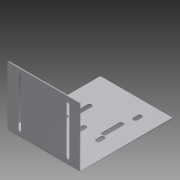
# Autodesk Inventor part: subframe
Saved by Autodesk Inventor 2014 SP2 (Build 180246200, 246)
## iProperties
Created: 2016-05-19
Part Number: subframe
Material: Aluminum 6061
Document SubType Name: Sheet Metal
Designer: cruiser
Density: 2.71 g/cm^3
Sheet Metal Rule: Default_mm
Appearance: Aluminum - Flat
Flat Pattern Width: 13.862 cm
Flat Pattern Length: 6.6 cm
Flat Pattern Area: 91.4895 cm^2
Sheet Metal Width: 138.620 mm
Sheet Metal Length: 66.000 mm
Sheet Metal Area: 9148.948 mm^2
Author: cruiser
Autodesk Inventor part; units mm, degrees
ref_plane "YZ Plane" through (0, 0, 0) normal (1, 0, 0) x (0, 1, 0)
ref_plane "XZ Plane" through (0, 0, 0) normal (0, 1, 0) x (-1, 0, 0)
ref_plane "XY Plane" through (0, 0, 0) normal (0, 0, 1) x (1, 0, 0)
sketch "Sketch1" plane through (0, 0, 0) normal (0, 1, 0) x (-1, 0, 0)
  line L0 (33, -27.5) -> (-33, -27.5)
  line L1 (-33, -27.5) -> (-33, 27.5)
  line L2 (-33, 27.5) -> (33, 27.5)
  line L3 (33, 27.5) -> (33, -27.5)
  line L4 (33, -27.5) -> (-33, 27.5) construction
  line L5 (-33, -27.5) -> (33, 27.5) construction
  point P0 (0, 0)
  dimension "d0" = 66
  dimension "d1" = 55
  measures "d0" distance of L1.end L2.end
  measures "d1" distance of L0.end L1.end
extrude "Plate1" add sketch "Sketch1" along normal blind 0.7937
sketch "Sketch3" plane through (0, 0.7937, 0) normal (0, 1, 0) x (1, 0, 0)
  line L0 (0, 0) -> (-33, 0)
  line L1 (-33, 0) -> (-33, 27.5)
  line L2 (-33, 27.5) -> (0, 27.5)
  line L3 (0, 27.5) -> (0, 0)
  circle A0 centre (-22, 16) radius 1.5
  circle A1 centre (-22, -16) radius 1.5
  circle A2 centre (22, 16) radius 1.5
  circle A3 centre (22, -16) radius 1.5
  line L4 (-22, 11) -> (-22, 21) construction
  line L5 (-20.5, 11) -> (-20.5, 21)
  line L6 (-23.5, 21) -> (-23.5, 11)
  arc A4 (-23.5, 11) -> (-20.5, 11) centre (-22, 11) ccw
  arc A5 (-20.5, 21) -> (-23.5, 21) centre (-22, 21) ccw
  line L7 (20.5, 11) -> (20.5, 21)
  line L8 (23.5, 21) -> (23.5, 11)
  arc A6 (20.5, 11) -> (23.5, 11) centre (22, 11) ccw
  arc A7 (23.5, 21) -> (20.5, 21) centre (22, 21) ccw
  line L9 (-20.5, -11) -> (-20.5, -21)
  line L10 (-23.5, -21) -> (-23.5, -11)
  arc A8 (-20.5, -11) -> (-23.5, -11) centre (-22, -11) ccw
  arc A9 (-23.5, -21) -> (-20.5, -21) centre (-22, -21) ccw
  arc A10 (20.5, -21) -> (23.5, -21) centre (22, -21) ccw
  line L11 (23.5, -21) -> (23.5, -11)
  line L12 (20.5, -11) -> (20.5, -21)
  arc A11 (23.5, -11) -> (20.5, -11) centre (22, -11) ccw
  line L13 (-23.5, 16) -> (-20.5, 16)
  line L14 (-20.5, 16) -> (-20.5, -16)
  line L15 (-20.5, -16) -> (-23.5, -16)
  line L16 (-23.5, -16) -> (-23.5, 16)
  line L17 (20.5, -16) -> (23.5, -16)
  line L18 (23.5, -16) -> (23.5, 16)
  line L19 (23.5, 16) -> (20.5, 16)
  line L20 (20.5, 16) -> (20.5, -16)
  dimension "d22" = 3
  dimension "d23" = 32
  dimension "d24" = 22
  dimension "d48" = 5
  dimension "d49" = 3
  constraints: 44 end point, 21 symmetric about line, 16 point on circle, 11 centre point, 8 parallel, 5 midpoint, 4 tangent, 3 horizontal, 3 perpendicular, 1 horizontal alignment, 11 other
  measures "d22" diameter of A0
  measures "d23" diameter of A0.centre L0
  measures "d24" distance from line of L3 A0.centre
  measures "d48" distance of A0.centre L4.end
  measures "d49" diameter of A5
extrude "Cut1" cut sketch "Sketch3" against normal blind 0.7937 contours L14 A8 L16 L0 | L0 L16 A4 L14 | A4 L6 A0 L5 | L9 A1 L10 A8 | L13 A0 | A0 L6 A5 L5 | A0 L13 | L15 A1 | L9 A9 L10 A1 | A1 L15 | L19 A2 | L8 A6 L7 A2 | A2 L7 A7 L8 | A2 L19 | L18 A11 L20 A6 | L11 A3 L12 A11 | L17 A3 | L11 A10 L12 A3 | A3 L17
sketch "Sketch2" plane through (-33, 0, -26.7063) normal (0, 0, -1) x (-1, 0, 0)
  line L0 (-66, 0) -> (0, 0)
  line L1 (0, 0) -> (0, 85)
  line L2 (0, 85) -> (-66, 85)
  line L3 (-66, 85) -> (-66, 0)
  constraints: 6 end point, 1 horizontal, 1 perpendicular, 1 vertical
edge flange "Flange1" height 70 angle 90 thickness 0.7937 bend radius 0.7937 thickness toward (0, 0, -1) relief tear relief width 0.7937 relief depth 0.3969 edges at (0, 0.7937, -27.5) wall of the first edge with corners at (33, 0, -26.7063) (-33, 0, -26.7063) (-33, 85, -26.7063) (33, 85, -26.7063)
bend "Bend1"
corner "Corner1"
sketch "Sketch4" plane through (33, 85, -27.5) normal (0, 0, -1) x (-1, 0, 0)
  line L0 (0, -83.4125) -> (66, -83.4125) projected
  line L1 (66, 0) -> (66, -83.4125) projected
  line L2 (0, 0) -> (66, 0) projected
  line L3 (33, -54) -> (33, -48) construction
  line L4 (35, -54) -> (35, -48)
  line L5 (31, -48) -> (31, -54)
  arc A0 (31, -54) -> (35, -54) centre (33, -54) ccw
  arc A1 (35, -48) -> (31, -48) centre (33, -48) ccw
  line L6 (33, -83.4125) -> (33, 0)
  line L7 (47.5, -44) -> (47.5, -28.5) construction
  line L8 (49.5, -44) -> (49.5, -28.5)
  line L9 (45.5, -28.5) -> (45.5, -44)
  arc A2 (45.5, -44) -> (49.5, -44) centre (47.5, -44) ccw
  arc A3 (49.5, -28.5) -> (45.5, -28.5) centre (47.5, -28.5) ccw
  line L10 (18.5, -44) -> (18.5, -28.5) construction
  line L11 (16.5, -44) -> (16.5, -28.5)
  line L12 (20.5, -28.5) -> (20.5, -44)
  arc A4 (16.5, -44) -> (20.5, -44) centre (18.5, -44) ccw
  arc A5 (20.5, -28.5) -> (16.5, -28.5) centre (18.5, -28.5) ccw
  line L13 (66, -85) -> (0, -85) projected
  line L14 (16, -50) -> (50, -50)
  line L15 (50, -50) -> (50, -16)
  line L16 (50, -16) -> (16, -16)
  line L17 (16, -16) -> (16, -50)
  circle A6 centre (16, -16) radius 2
  circle A7 centre (16, -50) radius 2
  circle A8 centre (50, -50) radius 2
  line L18 (33, -16) -> (33, -50)
  line L19 (16, -18) -> (16, -14) construction
  line L20 (18, -18) -> (18, -14)
  line L21 (14, -14) -> (14, -18)
  arc A9 (14, -18) -> (18, -18) centre (16, -18) ccw
  arc A10 (18, -14) -> (14, -14) centre (16, -14) ccw
  line L22 (16, -52) -> (16, -48) construction
  line L23 (18, -52) -> (18, -48)
  line L24 (14, -48) -> (14, -52)
  arc A11 (14, -52) -> (18, -52) centre (16, -52) ccw
  arc A12 (18, -48) -> (14, -48) centre (16, -48) ccw
  line L25 (50, -52) -> (50, -48) construction
  line L26 (52, -52) -> (52, -48)
  line L27 (48, -48) -> (48, -52)
  arc A13 (48, -52) -> (52, -52) centre (50, -52) ccw
  arc A14 (52, -48) -> (48, -48) centre (50, -48) ccw
  point P0 (33, -85)
  point P1 (33, -51)
  point P2 (47.5, -36.25)
  point P3 (18.5, -36.25)
  dimension "d25" = 3
  dimension "d26" = 4
  dimension "d29" = 4
  dimension "d30" = 15.5
  dimension "d31" = 14.5
  dimension "d46" = 48.75
  dimension "d47" = 34
  dimension "d50" = 34
  dimension "d51" = 34
  dimension "d52" = 4
  dimension "d53" = 4
  dimension "d54" = 4
  dimension "d55" = 35
  dimension "d56" = 0
  dimension "d57" = 2
  dimension "d58" = 4
  dimension "d59" = 2
  dimension "d60" = 4
  dimension "d61" = 2
  dimension "d62" = 4
  constraints: 60 end point, 24 point on circle, 20 tangent, 15 centre point, 9 midpoint, 9 parallel, 7 symmetric about line, 4 point on line, 3 coincident, 1 horizontal, 1 perpendicular, 2 other
  measures "d25" distance of point (33, -51) L3.end
  measures "d26" diameter of A1
  measures "d29" diameter of A3
  measures "d30" distance of L7.start L7.end
  measures "d31" distance from line of L6 point (47.5, -36.25)
  measures "d46" distance from line of point (47.5, -36.25) L13
  measures "d47" distance from line of L13 point (33, -51)
  measures "d50" distance of L16.end L15.end
  measures "d51" distance of L15.end L14.end
  measures "d52" diameter of A6
  measures "d53" diameter of A8
  measures "d54" diameter of A7
  measures "d55" distance between parallel lines of L13 L14
  measures "d56" distance between parallel lines of L18 L6
  measures "d57" distance of A6.centre L19.end
  measures "d58" diameter of A10
  measures "d59" distance of A7.centre L22.end
  measures "d60" diameter of A12
  measures "d61" distance of A8.centre L25.end
  measures "d62" diameter of A14
extrude "Cut2" cut sketch "Sketch4" against normal blind 0.7937 contours L6 L14 L4 A0 | A0 L5 L14 L6 | L14 L5 A1 L6 | L6 A1 L4 L14 | A7 L17 L14 | L14 L17 A7 | L23 A11 L24 A7 | A7 L17 A12 L23 | A8 L15 L14 | L27 A14 L15 A8 | L14 L15 A8 | A8 L26 A13 L27 | A6 L17 L16 | L16 L17 A6 | L20 A9 L17 A6 | A6 L21 A10 L20 | A7 L24 A12 L17 | L15 A14 L26 A8 | A6 L17 A9 L21 | A2 L9 A3 L8 | L11 A5 L12 A4
fillet "Corner Round1" radius 0.7937 4 edges at (-33, 0.3969, 27.5) (33, 0.3969, 27.5) (33, 85, -27.1031) (-33, 85, -27.1031)
equation "\"d0\" = subframe_x"
equation "\"d1\" = subframe_y"
equation "\"d22\" = m3_diameter"
equation "\"d23\" = 0.4 * frame_y"
equation "\"d24\" = 0.333333 * subframe_x"
equation "\"d49\" = m3_diameter"
equation "\"d20\" = Thickness"
equation "\"d26\" = m4_diameter"
equation "\"d29\" = m4_diameter"
equation "\"d33\" = Thickness"
equation "\"d3\" = BendReliefWidth"
equation "\"d4\" = BendReliefDepth"
equation "\"d5\" = MinimumRemnant"
equation "\"d6\" = BendRadius"
equation "\"d9\" = BendRadius"
equation "\"d11\" = CornerReliefSize"
equation "\"d12\" = GapSize"
equation "\"d13\" = JacobiRadiusSize"
equation "\"BendRadius\" = Thickness"
equation "\"BendReliefWidth\" = Thickness"
equation "\"BendReliefDepth\" = 0.5 * Thickness"
equation "\"CornerReliefSize\" = 4 * Thickness"
equation "\"MinimumRemnant\" = 2 * Thickness"
equation "\"TransitionRadius\" = BendRadius"
equation "\"JacobiRadiusSize\" = BendRadius"
equation "\"GapSize\" = Thickness"
equation "\"sm_thickness\" = 1.5875"
equation "\"very_thick_acrylic\" = 9.45"
equation "\"thick_acrylic\" = 5.88"
equation "\"thin_acrylic\" = 3.15"
equation "\"clear_acrylic\" = 3.15"
equation "\"wood_thickness\" = 6.72"
equation "\"m3_diameter\" = 3"
equation "\"m3_head\" = 6"
equation "\"m4_diameter\" = 4"
equation "\"m5_diameter\" = 5"
equation "\"m5_head\" = 10.3"
equation "\"brass_insert_drill\" = 4"
equation "\"m5_brass_insert_drill\" = 6.7"
equation "\"m3_press_nut_drill\" = 4.5"
equation "\"m5_press_nut_drill\" = 6.5"
equation "\"laser_body_diameter\" = 12"
equation "\"carrier_y\" = 251"
equation "\"carrier_z\" = 12"
equation "\"visor_x\" = 253.925"
equation "\"visor_y\" = 85.6"
equation "\"window_z\" = 332.225"
equation "\"window_y\" = 93.75"
equation "\"window_overlap\" = 48"
equation "\"acrylic_into_frame\" = 5"
equation "\"door_x\" = 251"
equation "\"door_z\" = 332.225"
equation "\"door_overlap\" = 48"
equation "\"linear_bearing_spacing\" = 198"
equation "\"tray_border\" = 25"
equation "\"bed_z\" = 25"
equation "\"crane_x\" = 223"
equation "\"crane_z2\" = 12"
equation "\"switch_spacing\" = 19"
equation "\"frame_top_z\" = 385"
equation "\"frame_bottom_z\" = 275"
equation "\"frame_total_z\" = 661.5875"
equation "\"frame_face_y\" = 45"
equation "\"frame_foot_z\" = 12"
equation "\"frame_screw_from_center\" = 25"
equation "\"laser_y_offset\" = 19.4"
equation "\"laser_diameter\" = 13"
equation "\"laser_z_offset\" = 55"
equation "\"laser_y\" = 15"
equation "\"laser_z\" = 75"
equation "\"laser_gap\" = 1"
equation "\"subframe_x\" = 66"
equation "\"subframe_y\" = 55"
equation "\"galvo_frame_x\" = 66"
equation "\"galvo_frame_z\" = 85"
equation "\"galvo_frame_y_offset\" = 27.5"
equation "\"drawer_x\" = 191.7875"
equation "\"drawer_y\" = 67.5"
equation "\"drawer_support_from_top\" = 48"
equation "\"drawer_screw_from_center\" = 55"
equation "\"nema17_x\" = 43"
equation "\"d2\" = BendRadius"
equation "\"d44\" = galvo_frame_x"
equation "\"al_thickness\" = 1.5875"
equation "\"rivet_diameter\" = 3.3"
equation "\"bend_factor\" = 2.26205"
equation "\"sm_bend\" = 3.591"
equation "\"al_bend\" = 3.591"
equation "\"frame_x\" = 353.375"
equation "\"carrier_z2\" = 25"
equation "\"carrier_y2\" = 76.825"
equation "\"injection_plastic\" = 3.15"
equation "\"handle_d\" = 4.7625"
equation "\"lmk8uu_shaft\" = 15"
equation "\"al2_bend\" = 3.591"
equation "\"al3_bend\" = 3.591"
equation "\"st2_thickness\" = 1.5875"
equation "\"st3_bend\" = 3.591"
equation "\"al1_bend\" = 1.7955"
equation "\"st2_bend\" = 3.591"
equation "\"st1_thickness\" = 0.79375"
equation "\"st3_thickness\" = 1.5875"
equation "\"al1_thickness\" = 0.79375"
equation "\"st1_bend\" = 1.7955"
equation "\"al3_thickness\" = 1.5875"
equation "\"acme_nut_d\" = 19.1"
equation "\"platform_upper_y\" = 46.625"
equation "\"frame_back_z\" = 498.2125"
equation "\"drawer_reservoir_overlap_x\" = 19.20625"
equation "\"acrylic1_thickness\" = 5.88"
equation "\"laserresin\" = 5"
equation "\"platform_fold_x\" = 25"
equation "\"crane_t\" = 1.5875"
equation "\"reservoir_t\" = 0.79375"
equation "\"platform_crane_gap\" = 0.1"
equation "\"al2_thickness\" = 1.5875"
equation "\"laser_holder_z\" = 75"
equation "\"crane_gap\" = 0.1"
equation "\"drawer_gap\" = 0.1"
equation "\"frame_gap\" = 0.1"
equation "\"acrylic3_thickness\" = 3.15"
equation "\"laser_holder_t\" = 0.79375"
equation "\"frame_back_y\" = 53.2125"
equation "\"foot_z\" = 15"
equation "\"drawer_t\" = 0.79375"
equation "\"frame_back_x\" = 268.2125"
equation "\"frame_back_t\" = 0.79375"
equation "\"frame_front_fold\" = 15"
equation "\"acme_nut_upper_d\" = 12.7"
equation "\"platform_t\" = 1.5875"
equation "\"tray_t\" = 5.88"
equation "\"foot_t\" = 0.79375"
equation "\"frame_front_y\" = 55"
equation "\"reservoir_flap_y\" = 20.79375"
equation "\"handle_hole_d\" = 5.0625"
equation "\"acrylic2_thickness\" = 3.15"
equation "\"drawer_fold\" = 15"
equation "\"handle_spacing\" = 50.8"
equation "\"frame_y\" = 80"
equation "\"Thickness\" = 0.79375"
body "Solid1"
